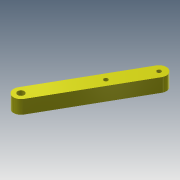
# Autodesk Inventor part: biela-dedo-1
Saved by Autodesk Inventor 2017 (Build 210142000, 142)
## iProperties
Created: 2018-05-30
Part Number: biela-dedo-1
Material: Generic
Document SubType Name: Modeling
Designer: Luiz Gustavo
Density: 1 g/cm^3
Appearance: Smooth - Yellow
Mass: 8.5918 g
Surface Area: 40.3163 cm^2
Volume: 8.5918 cm^3
Author: Luiz Gustavo
Autodesk Inventor part; units mm, degrees
ref_plane "YZ Plane" through (0, 0, 0) normal (1, 0, 0) x (0, 1, 0)
ref_plane "XZ Plane" through (0, 0, 0) normal (0, 1, 0) x (-1, 0, 0)
ref_plane "XY Plane" through (0, 0, 0) normal (0, 0, 1) x (1, 0, 0)
sketch "Sketch1" plane through (0, 0, 0) normal (0, 0, 1) x (1, 0, 0)
  line L0 (-64.4736, 0) -> (-50.2197, 25) construction
  line L1 (-64.4736, 0) -> (-87.28, -40) construction
  arc A0 (-82.502, -42.7242) -> (-92.0579, -37.2758) centre (-87.28, -40) ccw
  arc A1 (-54.9976, 27.7242) -> (-45.4417, 22.2758) centre (-50.2197, 25) ccw construction
  circle A2 centre (-50.2197, 25) radius 1.55
  circle A3 centre (-64.4736, 0) radius 1.55
  line L2 (-92.0579, -37.2758) -> (-54.9976, 27.7242)
  line L3 (-82.502, -42.7242) -> (-45.4417, 22.2758)
  arc A4 (-45.4417, 22.2758) -> (-54.9976, 27.7242) centre (-50.2197, 25) ccw
  arc A5 (-92.0579, -37.2758) -> (-82.502, -42.7242) centre (-87.28, -40) ccw
  point P0 (0, 0)
  dimension "d0" = 11
  dimension "d1" = 3.1
  constraints: 8 point on circle, 6 centre point, 4 coincident, 4 end point, 2 equal radius, 2 parallel, 2 tangent
  measures "d0" diameter of A0
  measures "d1" diameter of A2
extrude "Extrusion1" add sketch "Sketch1" along normal mid plane 10
sketch "Sketch2" plane through (0, 0, 0) normal (0, 0, 1) x (1, 0, 0)
  arc A0 (-92.0579, -37.2758) -> (-82.502, -42.7242) centre (-87.28, -40) ccw projected
  circle A1 centre (-87.28, -40) radius 2.5
  point P0 (0, 0)
  dimension "d4" = 5
  constraints: 1 centre point, 1 coincident
  measures "d4" diameter of A1
extrude "Extrusion2" cut sketch "Sketch2" along normal through all both and the other way through all
body "Solid1"
